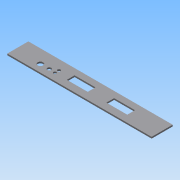
# Autodesk Inventor part: panel
Saved by Autodesk Inventor 2013 (Build 170138000, 138)
## iProperties
Created: 2014-07-23
Part Number: panel
Material: Generic
Document SubType Name: Sheet Metal
Designer: User
Density: 1 g/cm^3
Sheet Metal Rule: Default_mm
Author: User
Autodesk Inventor part; units mm, degrees
ref_plane "YZ Plane" through (0, 0, 0) normal (1, 0, 0) x (0, 1, 0)
ref_plane "XZ Plane" through (0, 0, 0) normal (0, 1, 0) x (-1, 0, 0)
ref_plane "XY Plane" through (0, 0, 0) normal (0, 0, 1) x (1, 0, 0)
sketch "Sketch1" plane through (0, 0, 0) normal (0, 0, 1) x (1, 0, 0)
  line L0 (-58.4821, 15.1494) -> (125.7179, 15.1494)
  line L1 (125.7179, 15.1494) -> (125.7179, -11.7506)
  line L2 (125.7179, -11.7506) -> (-58.4821, -11.7506)
  line L3 (-58.4821, -11.7506) -> (-58.4821, 15.1494)
  point P0 (0, 0)
  dimension "d0" = 184.2
  dimension "d2" = 26.9
  constraints: 8 end point, 2 parallel, 1 horizontal, 1 perpendicular
  measures "d0" distance of L0.start L0.end
  measures "d2" distance of L2.end L0.start
extrude "Extrusion1" add sketch "Sketch1" along normal blind 1.9
sketch "Sketch5" plane through (0, 0, 1.9) normal (0, 0, 1) x (1, 0, 0)
  line L0 (-58.4821, 15.1494) -> (-58.4821, -11.7506) projected
  line L1 (-58.4821, -11.7506) -> (125.7179, -11.7506) projected
  line L2 (125.7179, -11.7506) -> (125.7179, 15.1494) projected
  circle A0 centre (-25.9821, -2.0006) radius 3.5
  circle A1 centre (-14.7321, -2.0006) radius 2.5
  circle A2 centre (-6.9321, -2.5006) radius 1.9
  circle A3 centre (-6.9321, 2.6994) radius 1.9
  line L3 (8.5679, -2.7506) -> (35.1679, -2.7506)
  line L4 (35.1679, -2.7506) -> (35.1679, 7.1494)
  line L5 (35.1679, 7.1494) -> (8.5679, 7.1494)
  line L6 (8.5679, 7.1494) -> (8.5679, -2.7506)
  line L7 (59.0179, -2.7506) -> (85.6179, -2.7506)
  line L8 (85.6179, -2.7506) -> (85.6179, 7.1494)
  line L9 (85.6179, 7.1494) -> (59.0179, 7.1494)
  line L10 (59.0179, 7.1494) -> (59.0179, -2.7506)
  point P0 (0, 0)
  dimension "d56" = 7
  dimension "d58" = 5
  dimension "d59" = 32.5
  dimension "d60" = 43.75
  dimension "d61" = 9.75
  dimension "d62" = 9.75
  dimension "d63" = 3.8
  dimension "d64" = 3.8
  dimension "d65" = 51.55
  dimension "d66" = 51.55
  dimension "d67" = 9.25
  dimension "d68" = 14.45
  dimension "d69" = 26.6
  dimension "d70" = 26.6
  dimension "d71" = 9.9
  dimension "d72" = 9.9
  dimension "d73" = 9
  dimension "d74" = 9
  dimension "d75" = 117.15
  dimension "d76" = 66.7
  constraints: 16 end point, 4 centre point, 4 parallel, 2 horizontal, 2 perpendicular
  measures "d56" diameter of A0
  measures "d58" diameter of A1
  measures "d59" distance from line of A0.centre L0
  measures "d60" distance from line of A1.centre L0
  measures "d61" distance from line of A0.centre L1
  measures "d62" distance from line of A1.centre L1
  measures "d63" diameter of A2
  measures "d64" diameter of A3
  measures "d65" distance from line of A2.centre L0
  measures "d66" distance from line of A3.centre L0
  measures "d67" distance from line of A2.centre L1
  measures "d68" distance from line of A3.centre L1
  measures "d69" distance of L4.end L5.end
  measures "d70" distance of L8.end L9.end
  measures "d71" distance of L3.end L4.end
  measures "d72" distance of L7.end L8.end
  measures "d73" distance between parallel lines of L3 L1
  measures "d74" distance between parallel lines of L7 L1
  measures "d75" distance between parallel lines of L6 L2
  measures "d76" distance between parallel lines of L10 L2
extrude "Extrusion3" cut sketch "Sketch5" against normal through all
equation "\"BendRadius\" = Thickness"
equation "\"BendReliefWidth\" = Thickness"
equation "\"BendReliefDepth\" = 0.5 * Thickness"
equation "\"CornerReliefSize\" = 4 * Thickness"
equation "\"MinimumRemnant\" = 2 * Thickness"
equation "\"TransitionRadius\" = BendRadius"
equation "\"JacobiRadiusSize\" = BendRadius"
equation "\"GapSize\" = Thickness"
equation "\"Thickness\" = 0.5"
body "Solid1"
